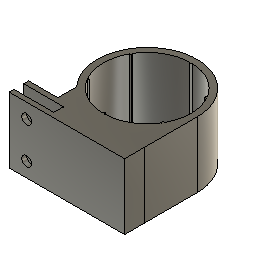
Fijador_arma (Autodesk Fusion 360 design; units mm, degrees)
Autodesk Fusion 360 part; units mm, degrees
sketch "Boceto1" plane through (0, 0, 0) normal (0, 0, 1) x (1, 0, 0)
  circle A0 centre (0, 0) radius 18
  circle A1 centre (0, 0) radius 17.5 construction
  line L0 (0, 0) -> (0, 17.25) construction
  line L1 (0, 17.25) -> (0.4301, 17.9949)
  line L2 (0, 17.25) -> (0.8601, 17.25) construction
  line L3 (0, 17.25) -> (-0.4301, 17.9949)
  line L4 (0, 17.25) -> (0.8601, 17.25) construction
  line L5 (-14.9389, 8.625) -> (-15.369, 9.3699)
  line L6 (-14.9389, 8.625) -> (-15.799, 8.625)
  line L7 (-14.9389, -8.625) -> (-15.799, -8.625)
  line L8 (-14.9389, -8.625) -> (-15.369, -9.3699)
  line L9 (0, -17.25) -> (-0.4301, -17.9949)
  line L10 (0, -17.25) -> (0.4301, -17.9949)
  line L11 (14.9389, -8.625) -> (15.369, -9.3699)
  line L12 (14.9389, -8.625) -> (15.799, -8.625)
  line L13 (14.9389, 8.625) -> (15.799, 8.625)
  line L14 (14.9389, 8.625) -> (15.369, 9.3699)
  circle A2 centre (0, 0) radius 20.5 construction
  line L15 (0, 0) -> (-19.792, 0) construction
  line L16 (0, 0) -> (0, -23.8) construction
  line L17 (0, -23.8) -> (16, -23.8) construction
  line L18 (0, -23.8) -> (-27, -23.8) construction
  line L19 (-19.792, 0) -> (-19.792, -23.8) construction
  line L20 (-19.792, -23.8) -> (-17.792, -23.8) construction
  line L21 (-19.792, -23.8) -> (-21.792, -23.8) construction
  arc A3 (20.5, 0) -> (-14.9826, -13.9918) centre (0, 0) ccw construction
  arc A4 (20.5, 0) -> (-14.9826, -13.9918) centre (0, 0) ccw
  line L22 (0, -23.8) -> (0, -27.8) construction
  line L23 (-14.9826, -13.9918) -> (-14.9826, -23.8) construction
  line L24 (-14.9826, -23.8) -> (-14.9826, -21.8) construction
  line L25 (-14.9826, -13.9918) -> (-14.9826, -21.8)
  line L26 (16, -23.8) -> (25, -23.8) construction
  line L27 (20.5, 0) -> (20.5, -23.8) construction
  line L28 (20.5, -23.8) -> (20.5, -21.8) construction
  line L29 (20.5, 0) -> (20.5, -21.8)
  line L30 (20.5, -21.8) -> (20.5, -27.8)
  line L31 (-14.9826, -21.8) -> (-27, -21.8)
  line L32 (20.5, -27.8) -> (20.5, -29.8)
  line L33 (-27, -21.8) -> (-27, -29.8)
  line L34 (-27, -29.8) -> (20.5, -29.8)
  dimension "d1" = 36
  dimension "d2" = 35
  dimension "d3" = 17.25
  dimension "d4" = 59.999
  dimension "d5" = 0.8601
  dimension "d6" = 120.001
  dimension "d7" = 0.8601
  dimension "d9" = 360
  dimension "d10" = 41
  dimension "d12" = 19.792
  dimension "d13" = 23.8
  dimension "d14" = 2
  dimension "d15" = 2
  dimension "d16" = 4
  dimension "d17" = 2
  dimension "d18" = 2
  dimension "d19" = 6
  dimension "d20" = 2
  dimension "d21" = 8
  constraint coincident A0.centre A1.centre
  constraint vertical L0
  constraint horizontal L2
  constraint coincident A0 L1.end
  constraint horizontal L4
  constraint perpendicular L0 L15
  constraint perpendicular L16 L17
  constraint perpendicular L16 L18
  constraint coincident L18 L19.end
  constraint perpendicular L18 L19
  constraint perpendicular L19 L20
  constraint perpendicular L19 L21
  constraint coincident A2 A3.end
  constraint perpendicular L17 L22
  constraint coincident L18 L23.end
  constraint perpendicular L18 L23
  constraint coincident L23 L24.end
  constraint parallel L17 L26
  constraint midpoint L26 L27.end
  constraint perpendicular L26 L28
  constraint perpendicular L26 L30
  constraint perpendicular L23 L31
  constraint perpendicular L17 L32
  constraint perpendicular L31 L33
  constraint perpendicular L32 L34
  measures "d1" diameter of A0
  measures "d2" diameter of A1
  measures "d3" distance of A0.centre L0.end
  measures "d4" angle of L1 L2
  measures "d5" distance of L0.end L1.end
  measures "d6" angle of L3 L4
  measures "d7" distance of L0.end L3.end
  measures "d10" diameter of A2
  measures "d12" distance of A0.centre L15.end
  measures "d13" distance of A0.centre L16.end
  measures "d14" distance of L19.end L20.end
  measures "d15" distance of L19.end L21.end
  measures "d16" distance of L16.end L22.end
  measures "d17" distance of L23.end L24.end
  measures "d18" distance of L27.end L28.end
  measures "d19" distance of L28.end L30.end
  measures "d20" distance of L30.end L32.end
  measures "d21" distance of L31.end L33.end
extrude "Extruir1" add sketch "Boceto1" along normal blind 27 contours A0 L13 L14 | A0 L11 L12 | A0 L1 L3 | A0 L9 L10 | A0 L5 L6 | A0 L7 L8 | A4 L25 L29 L30 L31 L32 L33 L34 makes body 1
sketch "Boceto2" plane through (0, -21.8, 0) normal (0, 1, 0) x (-1, 0, 0)
  line L0 (14.9826, 0) -> (27, 0)
  line L1 (27, 0) -> (27, 27)
  line L2 (27, 27) -> (14.9826, 27)
  line L3 (14.9826, 27) -> (14.9826, 0)
  line L4 (0, 0) -> (19.792, 0) construction
  line L5 (0, 0) -> (0, 13.5) construction
  line L6 (0, 13.5) -> (19.792, 13.5) construction
  line L7 (19.792, 0) -> (19.792, 6) construction
  line L8 (19.792, 6) -> (19.792, 21) construction
  circle A0 centre (19.792, 6) radius 2
  circle A1 centre (19.792, 21) radius 2
  dimension "d24" = 19.792
  dimension "d25" = 13.5
  dimension "d26" = 19.792
  dimension "d27" = 4
  dimension "d28" = 4
  constraint coincident L4.start L5.start
  constraint parallel L0 L4
  constraint perpendicular L4 L5
  constraint perpendicular L5 L6
  constraint perpendicular L6 L7
  constraint perpendicular L6 L8
  constraint coincident L7.end L8.start
  constraint coincident L8.end A1.centre
  measures "d24" distance of L4.start L4.end
  measures "d25" distance of L4.start L5.end
  measures "d26" distance of L5.end L6.end
  measures "d27" diameter of A0
  measures "d28" diameter of A1
extrude "Extruir2" cut sketch "Boceto2" against normal blind 8 contours A0 | A1 bodies 1
sketch "Sketch1" plane through (0, 0, 0) normal (0, 0, 1) x (1, 0, 0) in component "base_plate_doble_tranmision v25 v2"
  circle A0 centre (0, 0) radius 125
  line L0 (0, 0) -> (125, 0) construction
  line L1 (96, 34) -> (64, 34)
  line L2 (64, 34) -> (64, -34)
  line L3 (64, -34) -> (96, -34)
  line L4 (96, -34) -> (96, 34)
  line L5 (96, 34) -> (64, -34) construction
  line L6 (64, 34) -> (96, -34) construction
  line L7 (0, 0) -> (0, 125) construction
  line L8 (-64, 34) -> (-64, -34)
  line L9 (-64, -34) -> (-96, -34)
  line L10 (-96, 34) -> (-64, 34)
  line L11 (-96, -34) -> (-96, 34)
  line L12 (0, 0) -> (23, 0) construction
  line L13 (23, 0) -> (23, -20) construction
  line L14 (23, -20) -> (0, -20) construction
  line L15 (0, -20) -> (0, 0) construction
  circle A1 centre (23, -20) radius 1.5
  circle A2 centre (23, -20) radius 10 construction
  line L16 (23, -20) -> (33, -20) construction
  arc A3 (34.6057, -21.0154) -> (34.6057, -18.9846) centre (23, -20) ccw
  arc A4 (31.3182, -20.7278) -> (34.6057, -21.0154) centre (32.9619, -20.8716) ccw
  arc A5 (31.3182, -20.7278) -> (31.3182, -19.2722) centre (23, -20) ccw
  arc A6 (34.6057, -18.9846) -> (31.3182, -19.2722) centre (32.9619, -19.1284) ccw
  arc A7 (32.9619, -20.8716) -> (32.9619, -19.1284) centre (23, -20) ccw construction
  line L17 (23, -20) -> (32.9619, -19.1284) construction
  line L18 (23, -20) -> (32.9619, -20.8716) construction
  arc A8 (29.6822, -29.5431) -> (31.2378, -28.2378) centre (23, -20) ccw
  arc A9 (27.7894, -26.8399) -> (29.6822, -29.5431) centre (28.7358, -28.1915) ccw
  arc A10 (27.7894, -26.8399) -> (28.9043, -25.9043) centre (23, -20) ccw
  arc A11 (31.2378, -28.2378) -> (28.9043, -25.9043) centre (30.0711, -27.0711) ccw
  arc A12 (28.7358, -28.1915) -> (30.0711, -27.0711) centre (23, -20) ccw construction
  line L19 (28.7358, -28.1915) -> (23, -20) construction
  line L20 (30.0711, -27.0711) -> (23, -20) construction
  line L21 (23, -20) -> (29.4279, -27.6604) construction
  arc A13 (-31.3182, -19.2722) -> (-34.6057, -18.9846) centre (-32.9619, -19.1284) ccw
  arc A14 (-31.3182, -19.2722) -> (-31.3182, -20.7278) centre (-23, -20) ccw
  arc A15 (-34.6057, -18.9846) -> (-34.6057, -21.0154) centre (-23, -20) ccw
  arc A16 (-34.6057, -21.0154) -> (-31.3182, -20.7278) centre (-32.9619, -20.8716) ccw
  circle A17 centre (-23, -20) radius 1.5
  arc A18 (-28.9043, -25.9043) -> (-27.7894, -26.8399) centre (-23, -20) ccw
  arc A19 (-29.6822, -29.5431) -> (-27.7894, -26.8399) centre (-28.7358, -28.1915) ccw
  arc A20 (-28.9043, -25.9043) -> (-31.2378, -28.2378) centre (-30.0711, -27.0711) ccw
  arc A21 (-31.2378, -28.2378) -> (-29.6822, -29.5431) centre (-23, -20) ccw
  arc A22 (28.9043, -14.0957) -> (27.7894, -13.1601) centre (23, -20) ccw
  arc A23 (29.6822, -10.4569) -> (27.7894, -13.1601) centre (28.7358, -11.8085) ccw
  arc A24 (28.9043, -14.0957) -> (31.2378, -11.7622) centre (30.0711, -12.9289) ccw
  arc A25 (31.2378, -11.7622) -> (29.6822, -10.4569) centre (23, -20) ccw
  arc A26 (-27.7894, -13.1601) -> (-28.9043, -14.0957) centre (-23, -20) ccw
  arc A27 (-31.2378, -11.7622) -> (-28.9043, -14.0957) centre (-30.0711, -12.9289) ccw
  arc A28 (-29.6822, -10.4569) -> (-31.2378, -11.7622) centre (-23, -20) ccw
  arc A29 (-27.7894, -13.1601) -> (-29.6822, -10.4569) centre (-28.7358, -11.8085) ccw
  line L22 (19.5, 109) -> (-19.5, 109) construction
  line L23 (-19.5, 109) -> (-19.5, 99) construction
  line L24 (-19.5, 99) -> (19.5, 99) construction
  line L25 (19.5, 99) -> (19.5, 109) construction
  line L26 (19.5, 109) -> (-19.5, 99) construction
  line L27 (-19.5, 109) -> (19.5, 99) construction
  circle A30 centre (19.5, 104) radius 2
  circle A31 centre (-19.5, 104) radius 2
  circle A32 centre (0, 104) radius 15.5
  circle A33 centre (19.5, -104) radius 2
  circle A34 centre (-19.5, -104) radius 2
  circle A35 centre (0, -104) radius 15.5
  line L28 (15, 31.3397) -> (0, 57.3205)
  line L29 (0, 57.3205) -> (-15, 31.3397)
  line L30 (-15, 31.3397) -> (15, 31.3397)
  line L31 (-123.3896, -20) -> (-81.6662, 94.6342)
  line L32 (123.3896, -20) -> (81.6662, 94.6342)
  line L33 (-123.3896, -20) -> (123.3896, -20)
  line L34 (0, 75) -> (14, 75) construction
  circle A36 centre (14, 75) radius 1.5
  circle A37 centre (-14, 75) radius 1.5
  line L35 (0, 0) -> (14, 0) construction
  line L36 (14, 0) -> (14, 26) construction
  line L37 (14, 26) -> (0, 26) construction
  line L38 (0, 26) -> (0, 0) construction
  circle A38 centre (14, 26) radius 1.5
  circle A39 centre (-14, 26) radius 1.5
  line L39 (0, 0) -> (0, -65) construction
  line L40 (9.2, -58.5) -> (-9.2, -58.5) construction
  line L41 (-9.2, -58.5) -> (-9.2, -71.5) construction
  line L42 (-9.2, -71.5) -> (9.2, -71.5) construction
  line L43 (9.2, -71.5) -> (9.2, -58.5) construction
  line L44 (9.2, -58.5) -> (-9.2, -71.5) construction
  line L45 (-9.2, -58.5) -> (9.2, -71.5) construction
  circle A40 centre (9.2, -58.5) radius 1.5
  circle A41 centre (-9.2, -58.5) radius 1.5
  circle A42 centre (-9.2, -71.5) radius 1.5
  circle A43 centre (9.2, -71.5) radius 1.5
  circle A44 centre (33, -20) radius 1.5
  line L46 (23, -20) -> (29.4279, -12.3396) construction
  circle A45 centre (29.4279, -12.3396) radius 1.5
  circle A46 centre (29.4279, -27.6604) radius 1.5
  circle A47 centre (-29.4279, -12.3396) radius 1.5
  circle A48 centre (-33, -20) radius 1.5
  circle A49 centre (-29.4279, -27.6604) radius 1.5
  line L47 (-50, 66) -> (-30, 66) construction
  circle A50 centre (-30, 66) radius 1.5
  circle A51 centre (-50, 66) radius 1.5
  circle A52 centre (30, 66) radius 1.5
  circle A53 centre (50, 66) radius 1.5
  line L48 (45, -70) -> (55, -70) construction
  circle A54 centre (55, -70) radius 1.5
  circle A55 centre (45, -70) radius 1.5
  circle A56 centre (-45, -70) radius 1.5
  circle A57 centre (-55, -70) radius 1.5
  line L49 (-80, -34) -> (-120.2872, -34)
  line L50 (80, -34) -> (120.2872, -34)
  line L51 (80, 34) -> (120.2872, 34)
  line L52 (-80, 34) -> (-120.2872, 34)
  line L53 (80, -34) -> (80, -96.0469)
  line L54 (-96, -34) -> (-96, -80.0562)
  line L55 (-80, -34) -> (-80, -96.0469)
  line L56 (80, 34) -> (80, 96.0469)
  line L57 (-80, 34) -> (-80, 96.0469)
  line L58 (80, 34) -> (-80, 34)
  line L59 (70, -50) -> (-70, -50) construction
  line L60 (-70, -50) -> (-70, -90) construction
  line L61 (-70, -90) -> (70, -90) construction
  line L62 (70, -90) -> (70, -50) construction
  line L63 (70, -50) -> (-70, -90) construction
  line L64 (-70, -50) -> (70, -90) construction
  circle A58 centre (-70, -90) radius 2
  circle A59 centre (-70, -50) radius 2
  circle A60 centre (70, -50) radius 2
  circle A61 centre (70, -90) radius 2
  line L65 (64, 34) -> (64, 107.3732)
  line L66 (-64, 34) -> (-64, 107.3732)
  line L67 (23, -20) -> (23, 55) construction
  circle A62 centre (23, 55) radius 1.5
  circle A63 centre (23, 55) radius 10 construction
  line L68 (23, 55) -> (33, 55) construction
  line L69 (23, 55) -> (29.4279, 62.6604) construction
  circle A64 centre (29.4279, 62.6604) radius 1.5
  circle A65 centre (33, 55) radius 1.5
  circle A66 centre (29.4279, 47.3396) radius 1.5
  circle A67 centre (-29.4279, 62.6604) radius 1.5
  circle A68 centre (-23, 55) radius 1.5
  circle A69 centre (-33, 55) radius 1.5
  circle A70 centre (-29.4279, 47.3396) radius 1.5
  line L70 (-59.3717, 110) -> (59.3717, 110)
  line L71 (93, -34) -> (93, -83.5225)
  line L72 (-93, -34) -> (-93, -83.5225)
  line L73 (0, -65) -> (15, -65) construction
  line L74 (24.2, -58.5) -> (5.8, -58.5) construction
  line L75 (5.8, -58.5) -> (5.8, -71.5) construction
  line L76 (5.8, -71.5) -> (24.2, -71.5) construction
  line L77 (24.2, -71.5) -> (24.2, -58.5) construction
  line L78 (24.2, -58.5) -> (5.8, -71.5) construction
  line L79 (5.8, -58.5) -> (24.2, -71.5) construction
  circle A71 centre (24.2, -58.5) radius 1.5
  circle A72 centre (5.8, -58.5) radius 1.5
  circle A73 centre (5.8, -71.5) radius 1.5
  circle A74 centre (24.2, -71.5) radius 1.5
  circle A75 centre (-5.8, -58.5) radius 1.5
  circle A76 centre (-5.8, -71.5) radius 1.5
  circle A77 centre (-24.2, -58.5) radius 1.5
  circle A78 centre (-24.2, -71.5) radius 1.5
  line L80 (0, -30) -> (5, -30) construction
  circle A79 centre (5, -30) radius 1.5
  circle A80 centre (-5, -30) radius 1.5
  line L81 (5, -30) -> (-5, -30) construction
  line L82 (-5, -30) -> (-5, -5) construction
  line L83 (-5, -5) -> (5, -5) construction
  line L84 (5, -5) -> (5, -30) construction
  circle A81 centre (-5, -5) radius 1.5
  circle A82 centre (5, -5) radius 1.5
  line L85 (0, 100) -> (-50, 100) construction
  circle A83 centre (-50, 100) radius 2
  circle A84 centre (50, 100) radius 2
  point P0 (80, 0)
  point P1 (0, 104)
  point P2 (0, 40)
  point P3 (0, -65)
  point P4 (50, -70)
  point P5 (0, -70)
  point P6 (-10, 82)
  point P7 (15, -65)
  dimension "d1_1" = 32
  dimension "d2_1" = 68
  dimension "d5_1" = 250
  dimension "d6_1" = 80
  dimension "d7_1" = 20
  dimension "d8_1" = 23
  dimension "d9_1" = 3
  dimension "d10_1" = 20
  dimension "d11" = 1.65
  dimension "d12_1" = 5
  dimension "d13_1" = 5
  dimension "d14_1" = 10
  dimension "d15_1" = 50
  dimension "d16_1" = 4
  dimension "d17_1" = 4
  dimension "d18_1" = 39
  dimension "d19_1" = 10
  dimension "d20_1" = 104
  dimension "d21_1" = 31
  dimension "d22_1" = 40
  dimension "d23_1" = 30
  dimension "d26_1" = 40
  dimension "d27_1" = 20
  dimension "d28_1" = 14
  dimension "d29_1" = 3
  dimension "d30_1" = 75
  dimension "d31" = 3
  dimension "d32" = 14
  dimension "d33" = 49
  dimension "d34" = 18.4
  dimension "d35" = 13
  dimension "d36" = 3
  dimension "d38" = 65
  dimension "d39" = 3
  dimension "d40" = 50
  dimension "d41" = 3
  dimension "d42" = 3
  dimension "d45" = 3
  dimension "d46" = 3
  dimension "d47" = 20
  dimension "d48" = 66
  dimension "d49" = 30
  dimension "d50" = 3
  dimension "d51" = 3
  dimension "d52" = 10
  dimension "d53" = 70
  dimension "d54" = 50
  dimension "d61" = 50
  dimension "d63" = 4
  dimension "d65" = 140
  dimension "d66" = 40
  dimension "d67" = 75
  dimension "d68" = 3
  dimension "d69" = 20
  dimension "d70" = 50
  dimension "d71" = 3
  dimension "d72" = 3
  dimension "d73" = 110
  dimension "d74" = 13
  dimension "d80" = 10
  dimension "d81" = 82
  dimension "d84" = 18.4
  dimension "d85" = 13
  dimension "d86" = 3
  dimension "d87" = 15
  dimension "d90" = 3
  dimension "d91" = 5
  dimension "d92" = 30
  dimension "d93" = 25
  dimension "d94" = 4
  dimension "d95" = 50
  dimension "d96" = 100
  constraint coincident A0.centre L0.start
  constraint coincident A0 L0.end
  constraint horizontal L0
  constraint horizontal L1
  constraint perpendicular L1 L2
  constraint parallel L1 L3
  constraint parallel L2 L4
  constraint coincident L5 P0
  constraint coincident L6 P0
  constraint coincident L0 P0
  constraint coincident A0 L7.end
  constraint perpendicular L0 L7
  constraint symmetric L1.start L7 L10.start
  constraint symmetric L1.end L7 L8.start
  constraint symmetric L2.end L7 L8.end
  constraint symmetric L3.end L7 L9.end
  constraint horizontal L12
  constraint vertical L13
  constraint horizontal L14
  constraint vertical L15
  constraint coincident L13.end L14.start
  constraint concentric A1 A2
  constraint coincident A2 L16.end
  constraint perpendicular L13 L16
  constraint tangent A3 A4
  constraint tangent A4 A5
  constraint tangent A5 A6
  constraint tangent A3 A6
  constraint coincident A2 A6.centre
  constraint coincident A6.centre A7.end
  constraint coincident A4.centre A7.start
  constraint tangent A8 A9
  constraint tangent A9 A10
  constraint tangent A10 A11
  constraint tangent A8 A11
  constraint coincident A2 A11.centre
  constraint equal A3 A8
  constraint coincident A9.centre A12.start
  constraint coincident A11.centre A12.end
  constraint midpoint A12 L21.end
  constraint symmetric L7 A1 A17
  constraint symmetric L7 A3.end A13.end
  constraint symmetric L7 A3.start A15.end
  constraint symmetric L7 A4.start A14.end
  constraint symmetric L7 A5.end A13.start
  constraint symmetric L7 A3 A15
  constraint symmetric L7 A4 A16
  constraint symmetric L7 A5 A14
  constraint symmetric L7 A6 A13
  constraint symmetric L7 A8.end A20.end
  constraint symmetric L7 A8.start A19.start
  constraint symmetric L7 A9.start A18.end
  constraint symmetric L7 A10.end A18.start
  constraint symmetric L7 A8 A21
  constraint symmetric L7 A9 A19
  constraint symmetric L7 A10 A18
  constraint symmetric L7 A11 A20
  constraint symmetric L14 A8.end A24.end
  constraint symmetric L14 A8.start A23.start
  constraint symmetric L14 A9.start A22.end
  constraint symmetric L14 A10.end A22.start
  constraint symmetric L14 A8 A25
  constraint symmetric L14 A9 A23
  constraint symmetric L14 A10 A22
  constraint symmetric L14 A11 A24
  constraint symmetric L14 A18.end A26.start
  constraint symmetric L14 A18.start A26.end
  constraint symmetric L14 A18 A26
  constraint symmetric L14 A19.start A28.start
  constraint symmetric L14 A19 A29
  constraint symmetric L14 A20.end A27.start
  constraint symmetric L14 A20 A27
  constraint symmetric L14 A21 A28
  constraint horizontal L22
  constraint perpendicular L22 L23
  constraint parallel L22 L24
  constraint parallel L23 L25
  constraint coincident L26 P1
  constraint coincident L27 P1
  constraint coincident L7 P1
  constraint midpoint L25 A30.centre
  constraint midpoint L23 A31.centre
  constraint coincident P1 A32.centre
  constraint symmetric L0 A30 A33
  constraint symmetric L0 A31 A34
  constraint symmetric L0 A32 A35
  constraint coincident L7 P2
  constraint horizontal L30
  constraint coincident A0 L31.start
  constraint coincident A0 L31.end
  constraint symmetric L7 L31.start L32.start
  constraint symmetric L7 L31.end L32.end
  constraint coincident L7 L34.start
  constraint perpendicular L7 L34
  constraint coincident L34.end A36.centre
  constraint symmetric L7 A36 A37
  constraint horizontal L35
  constraint vertical L36
  constraint horizontal L37
  constraint vertical L38
  constraint coincident L36.end L37.start
  constraint symmetric L38 A38 A39
  constraint perpendicular L35 L39
  constraint horizontal L40
  constraint perpendicular L40 L41
  constraint parallel L40 L42
  constraint parallel L41 L43
  constraint coincident L44 P3
  constraint coincident L45 P3
  constraint coincident P3 L39.end
  constraint coincident L40.start L43.end
  constraint coincident L40.end L41.start
  constraint coincident L41.end L42.start
  constraint coincident L42.end L43.start
  constraint equal A40 A41
  constraint equal A40 A42
  constraint equal A40 A43
  constraint coincident L16.end A44.centre
  constraint coincident A2 L46.end
  constraint coincident L46.end A45.centre
  constraint coincident L21.end A46.centre
  constraint symmetric L39 A44 A48
  constraint symmetric L39 A45 A47
  constraint symmetric L39 A46 A49
  constraint horizontal L47
  constraint coincident L47.end A50.centre
  constraint coincident L47.start A51.centre
  constraint symmetric L7 A50 A52
  constraint symmetric L7 A51 A53
  constraint horizontal L48
  constraint coincident L48.end A54.centre
  constraint coincident L48.start A55.centre
  constraint midpoint L48 P4
  constraint symmetric L7 A54 A57
  constraint symmetric L7 A55 A56
  constraint midpoint L9 L49.start
  constraint coincident A0 L49.end
  constraint perpendicular L36 L49
  constraint midpoint L3 L50.start
  constraint coincident A0 L50.end
  constraint parallel L3 L50
  constraint midpoint L1 L51.start
  constraint coincident A0 L51.end
  constraint parallel L1 L51
  constraint midpoint L10 L52.start
  constraint coincident A0 L52.end
  constraint perpendicular L8 L52
  constraint coincident A0 L53.end
  constraint perpendicular L50 L53
  constraint coincident A0 L54.end
  constraint perpendicular L9 L54
  constraint coincident A0 L55.end
  constraint perpendicular L9 L55
  constraint coincident A0 L56.end
  constraint perpendicular L51 L56
  constraint coincident A0 L57.end
  constraint perpendicular L10 L57
  constraint horizontal L59
  constraint perpendicular L59 L60
  constraint parallel L59 L61
  constraint parallel L60 L62
  constraint coincident L63 P5
  constraint coincident L64 P5
  constraint coincident L39 P5
  constraint coincident L60.end L61.start
  constraint coincident L59.end L60.start
  constraint coincident L59.start L62.end
  constraint coincident L61.end L62.start
  constraint equal A58 A59
  constraint equal A59 A61
  constraint equal A59 A60
  constraint coincident A0 L65.end
  constraint perpendicular L58 L65
  constraint coincident A0 L66.end
  constraint perpendicular L10 L66
  constraint parallel L13 L67
  constraint coincident L67.end A62.centre
  constraint concentric A62 A63
  constraint coincident A63 L68.end
  constraint perpendicular L67 L68
  constraint coincident A63 L69.end
  constraint coincident L69.end A64.centre
  constraint coincident L68.end A65.centre
  constraint symmetric L68 A64 A66
  constraint symmetric L7 A62 A68
  constraint symmetric L7 A64 A67
  constraint symmetric L7 A65 A69
  constraint symmetric L7 A66 A70
  constraint coincident A0 L70.start
  constraint coincident A0 L70.end
  constraint parallel L24 L70
  constraint coincident L50 L71.start
  constraint coincident A0 L71.end
  constraint perpendicular L50 L71
  constraint symmetric L7 L71.start L72.start
  constraint symmetric L7 L71.end L72.end
  constraint horizontal L73
  constraint horizontal L74
  constraint perpendicular L74 L75
  constraint parallel L74 L76
  constraint parallel L75 L77
  constraint coincident L78 P7
  constraint coincident L79 P7
  constraint coincident P7 L73.end
  constraint coincident L74.start L77.end
  constraint coincident L74.end L75.start
  constraint coincident L75.end L76.start
  constraint coincident L76.end L77.start
  constraint equal A71 A72
  constraint equal A71 A73
  constraint equal A71 A74
  constraint symmetric L39 A71 A77
  constraint symmetric L39 A72 A75
  constraint symmetric L39 A73 A76
  constraint symmetric L39 A74 A78
  constraint coincident L7 L80.start
  constraint perpendicular L7 L80
  constraint coincident L80.end A79.centre
  constraint symmetric L7 A79 A80
  constraint horizontal L81
  constraint vertical L82
  constraint horizontal L83
  constraint vertical L84
  constraint coincident A80.centre L82
  constraint coincident L82.end L83.start
  constraint coincident L83.end L84.start
  constraint equal A79 A81
  constraint equal A79 A82
  constraint coincident L7 L85.start
  constraint perpendicular L7 L85
  constraint coincident L85.end A83.centre
  constraint symmetric L7 A83 A84
  measures "d1_1" distance of L2.end L3.end
  measures "d2_1" distance of L1.start L3.end
  measures "d5_1" diameter of A0
  measures "d6_1" distance of A0.centre P0
  measures "d7_1" distance of L12.end L13.end
  measures "d8_1" distance of L13.end L14.end
  measures "d9_1" diameter of A1
  measures "d10_1" diameter of A2
  measures "d11" radius of A6
  measures "d12_1" angle of L16 L17
  measures "d13_1" angle of L16 L18
  measures "d14_1" angle of L19 L20
  measures "d15_1" angle of L16 L21
  measures "d16_1" diameter of A31
  measures "d17_1" diameter of A30
  measures "d18_1" distance of L23.end L24.end
  measures "d19_1" distance of L22.start L24.end
  measures "d20_1" distance of A0.centre A32.centre
  measures "d21_1" diameter of A32
  measures "d22_1" distance of A0.centre P2
  measures "d23_1" distance of L28.start L28.end
  measures "d26_1" angle of L31 L32
  measures "d27_1" distance of A0.centre L33
  measures "d28_1" distance of L34.start L34.end
  measures "d29_1" diameter of A36
  measures "d30_1" distance of A0.centre L34
  measures "d31" diameter of A38
  measures "d32" distance of L36.end L37.end
  measures "d33" distance of L34.end L37
  measures "d34" distance of L41.end L42.end
  measures "d35" distance of L40.end L41.end
  measures "d36" diameter of A40
  measures "d38" distance of A0.centre P3
  measures "d39" diameter of A44
  measures "d40" angle of L33 L46
  measures "d41" diameter of A45
  measures "d42" diameter of A46
  measures "d45" diameter of A50
  measures "d46" diameter of A51
  measures "d47" distance of L47.start L47.end
  measures "d48" distance of A0.centre L47
  measures "d49" distance of L7 L47.end
  measures "d50" diameter of A54
  measures "d51" diameter of A55
  measures "d52" distance of L48.start L48.end
  measures "d53" distance of L0 L48
  measures "d54" horizontal distance of A0.centre P4
  measures "d61" distance of A0.centre L59
  measures "d63" diameter of A59
  measures "d65" distance of L60.end L61.end
  measures "d66" distance of L59.start L61.end
  measures "d67" distance of L13.end L67.end
  measures "d68" diameter of A62
  measures "d69" diameter of A63
  measures "d70" angle of L68 L69
  measures "d71" diameter of A64
  measures "d72" diameter of A65
  measures "d73" distance of A0.centre L70
  measures "d74" distance of L53 L71
  measures "d80" distance of L7 P6
  measures "d81" vertical distance of A0.centre P6
  measures "d84" distance of L75.end L76.end
  measures "d85" distance of L74.end L75.end
  measures "d86" diameter of A71
  measures "d87" distance of P3 P7
  measures "d90" diameter of A79
  measures "d91" distance of L80.start L80.end
  measures "d92" distance of A0.centre L80
  measures "d93" distance of A80.centre L82.end L18
  measures "d94" diameter of A83
  measures "d95" distance of L85.start L85.end
  measures "d96" distance of A0.centre L85
extrude "Extrude1" add sketch "Sketch1" against normal blind 4 separate body contours A0 L3 L50 L53 L71 | L2 L8 A1 A3 A5 A6 A13 A14 A15 A17 L28 L29 L30 L33 L58 | A0 L2 L3 L8 L9 A1 A3 A4 A5 A14 A15 A16 A17 L33 L53 L55 | A0 A32 L28 L29 L58 L65 L66 L70 | A3 A5 A6 L33 A44 | A3 A4 A5 L33 A44 | A0 L9 L49 L55 L72 | L28 L29 L58 | L28 L29 L30 L58 | A32 L70 | A14 A15 A16 L33 A48 | A13 A14 A15 L33 A48 | A8 A9 A10 A11 | A18 A19 A20 A21 | A22 A23 A24 A25 | A26 A27 A28 A29 | A40 | A41 | A42 | A43 | A50 | A51 | A52 | A53 picked at (1.4689, 102.3391) makes body 2 in component "base_plate_doble_tranmision v25 v2"
fillet "Fillet4" radius 6.35 4 edges at (64, -34, -2) (93, -34, -2) (-93, -34, -2) (-64, -34, -2) on bodies 2 in component "base_plate_doble_tranmision v25 v2"
move_body "Desplazar1" bodies 2 to x (1, 0, 0) y (0, 0, -1) z (0, 1, 0) at (0, -121, -129) in component "base_plate_doble_tranmision v25 v2"
move_body "Desplazar2" bodies 2 to x (1, 0, 0) y (0, 1, 0) z (0, 0, 1) at (-120, 0, 0) in component "base_plate_doble_tranmision v25 v2"
combine "Combinar1" operation cut target body 1 tool bodies 2 body 2 seen with x (0, 0, -1) y (0, 1, 0) z (1, 0, 0) at (19.1585, 97.1611, -168.9575)
delete_face "SuprimirCaras1" 1 faces at (-21.6033, -26.5055, 20.096) on bodies 1
component "base_plate_doble_tranmision v25 v2" placed x (0, 0, -1) y (0, 1, 0) z (1, 0, 0) at (19.1585, 97.1611, -168.9575)
equation "d13_1 = d12_1"
equation "d17_1 = d16_1"
equation "d28_1 = ( 28 / 2 ) * 1 mm"
